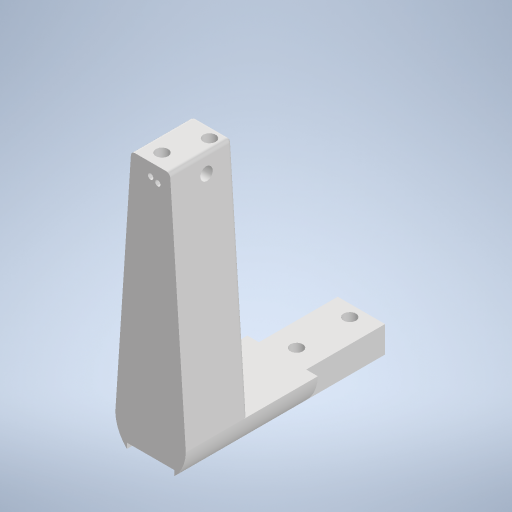
# Autodesk Inventor part: microstim_holder_bottom
Saved by Autodesk Inventor 2024 (Build 280153000, 153)
## iProperties
Created: 2023-05-03
Part Number: microstim_holder_bottom
Material: Generic
Document SubType Name: Modeling
Designer: Rober
Mass: 538.313 g
Surface Area: 676.575 cm^2
Volume: 538.313 cm^3
Density: 1 g/cm^3
Appearance: Default
Author: Rober
Autodesk Inventor part; units mm, degrees
ref_plane "YZ Plane" through (0, 0, 0) normal (1, 0, 0) x (0, 1, 0)
ref_plane "XZ Plane" through (0, 0, 0) normal (0, 1, 0) x (-1, 0, 0)
sketch "Sketch1" plane through (0, 0, 0) normal (0, 1, 0) x (-1, 0, 0)
  line L0 (3.05, -5.3255) -> (-3.05, -5.3255)
  line L1 (-3.05, -5.3255) -> (-3.05, 4.8245)
  line L2 (-3.05, 4.8245) -> (3.05, 4.8245)
  line L3 (3.05, 4.8245) -> (3.05, -5.3255)
  line L4 (0.925, 4.8245) -> (-0.925, 4.8245)
  line L5 (0.925, 4.8245) -> (0.925, -5.3255)
  line L6 (-0.925, 4.8245) -> (-0.925, -5.3255)
  circle A0 centre (0, 3.0245) radius 0.8
  circle A1 centre (0, -3.8255) radius 0.8
  line L7 (0, 4.8245) -> (0, -5.3255)
  line L8 (-3.05, 0) -> (3.05, 0)
  point P0 (0, 0)
  dimension "d13" = 6.1
  dimension "d44" = 1.85
  dimension "d45" = 2.125
  dimension "d46" = 1.6
  dimension "d47" = 1.6
  dimension "d128" = 6.85
  constraints: 18 end point, 9 point on line, 4 perpendicular, 3 midpoint, 2 centre point, 2 parallel, 1 horizontal
  measures "d13" distance of L0.start L0.end
  measures "d44" distance of L4.start L4.end
  measures "d45" distance from line of L3 L4.start
  measures "d46" diameter of A0
  measures "d47" diameter of A1
  measures "d128" distance of A0.centre A1.centre
extrude "Extrusion1" add sketch "Sketch1" along normal blind 3.4 contours L0 L5 L8 L3 | L0 L7 A1 L8 L5 | L8 L5 L2 L3 | L0 L6 L8 L7 A1 | L8 L7 A0 L2 L5 | L0 L1 L8 L6 | L8 L6 L2 L7 A0 | L8 L1 L2 L6
extrude "Extrusion6" add sketch "Sketch1" against normal blind 1 contours L0 L7 A1 L8 L5 | L0 L6 L8 L7 A1 | L8 L7 A0 L2 L5 | L8 L6 L2 L7 A0
sketch "Sketch13" plane through (-3.05, 3.4, 4.8245) normal (0, 0, 1) x (1, 0, 0)
  line L0 (0, 0) -> (0, -2.7)
  line L1 (0, -3.4) -> (0, 0) projected
  line L2 (0, -2.7) -> (6.1, -2.7)
  line L3 (6.1, -3.4) -> (6.1, 0) projected
  line L4 (6.1, 0) -> (6.1, -2.7)
  line L5 (0, 0) -> (6.1, 0)
  arc A0 (-1.4899, 0) -> (0, -3.4) centre (3.4689, 0.1465) ccw
  line L6 (-1.4899, 0) -> (12.0323, 0)
  line L7 (2.25, 0) -> (3.85, 0) projected
  line L8 (3.05, 0) -> (3.05, -3.4)
  line L9 (3.05, 0) -> (3.05, -3.4)
  arc A1 (6.1, -3.4) -> (7.5899, 0) centre (2.6311, 0.1465) ccw
  point P0 (6.1, -3.41)
  point P1 (7.5899, 0)
  dimension "d56" = 2.7
  constraints: 14 end point, 6 point on circle, 3 perpendicular, 2 centre point, 2 point on line, 2 symmetric about line, 1 collinear, 1 horizontal, 1 midpoint, 1 vertical, 1 other
  measures "d56" distance of L0.start L0.end
extrude "Extrusion8" add sketch "Sketch13" along normal blind 17
ref_plane "Work Plane3" through (-3.05, 3.4, 13.8245) normal (0, 0, 1) x (1, 0, 0)
sketch "Sketch29" plane through (-3.05, 3.4, 13.8245) normal (0, 0, 1) x (1, 0, 0)
  line L0 (3.85, -4.4) -> (2.25, -4.4) projected
  line L1 (3.05, -4.4) -> (3.05, 30.1)
  line L2 (5.55, 30.1) -> (3.05, 30.1)
  line L3 (3.05, 30.1) -> (0.55, 30.1)
  line L4 (5.55, 30.1) -> (7.5899, 0)
  line L5 (0.55, 30.1) -> (-1.4899, 0)
  line L6 (0, 0) -> (6.1, 0)
  line L7 (0, 0) -> (-1.4899, 0) projected
  line L8 (6.1, 0) -> (0, 0) projected
  line L9 (-1.4899, 0) -> (7.5899, 0)
  line L10 (-1.4899, 0) -> (7.5899, 0)
  point P0 (3.05, -3.4)
  point P1 (3.0506, 28.6)
  point P2 (3.05, 0)
  point P3 (3.05, 0)
  dimension "d137" = 34.5
  dimension "d156" = 2.5
  constraints: 17 end point, 3 collinear, 3 horizontal, 1 coincident, 1 midpoint, 1 vertical
  measures "d137" distance of L1.start L1.end
  measures "d156" distance of L2.start L1.end
extrude "Extrusion20" add sketch "Sketch29" along normal blind 8
fillet "Fillet6" radius 0.5 2 edges at (3.5199, 18.45, 13.8245) (-3.5199, 18.45, 13.8245)
sketch "Sketch24" plane through (-3.05, 0, -5.3255) normal (-1, 0, 0) x (0, 0, 1)
  circle A0 centre (22.5969, 31.2712) radius 0.8
  point P0 (5.3255, 0)
  point P1 (27.15, 0.7)
  dimension "d109" = 1.6
  constraints: 1 centre point
  measures "d109" diameter of A0
sketch "Sketch31" plane through (-3.05, 3.4, 13.8245) normal (0, 0, -1) x (-1, 0, 0)
  line L0 (-3.05, -3.4) -> (-3.05, 28.5)
  circle A0 centre (-3.05, 28.5) radius 0.355
  circle A1 centre (-3.9848, 28.2193) radius 0.355
  circle A2 centre (-3.9848, 28.2193) radius 0.3556 projected
  dimension "d145" = 31.9
  dimension "d147" = 0.71
  dimension "d155" = 0.71
  constraints: 2 centre point, 2 coincident, 2 end point, 1 vertical
  measures "d145" distance of L0.start L0.end
  measures "d147" diameter of A0
  measures "d155" diameter of A1
extrude "Extrusion22" cut sketch "Sketch31" against normal through all
fillet "Fillet7" radius 0.5 4 edges at (-2.5, 33.5, 18.0745) (2.3532, 33.5, 13.9709) (0, 33.5, 13.8245) (2.5, 33.5, 18.0745)
extrude "Extrusion24" cut sketch "Sketch24" against normal through all
sketch "Sketch35" plane through (-2.0327, 33.5, 21.8245) normal (0, 1, 0) x (1, 0, 0)
  circle A0 centre (3.1617, 6.4619) radius 0.8
  circle A1 centre (1.7036, 1.8035) radius 0.8
  point P0 (2.0327, 21.8245)
  dimension "d159" = 1.6
  dimension "d160" = 1.6
  constraints: 2 centre point
  measures "d159" diameter of A0
  measures "d160" diameter of A1
extrude "Extrusion25" cut sketch "Sketch35" against normal blind 1.5
equation "\"d13\" = base_width"
equation "\"d45\" = -0.5 * d44 + 0.5 * d13"
equation "\"d4\" = base_length"
equation "\"base_width\" = 6.1"
equation "\"base_length\" = 3.4"
equation "\"base_screw_diameter\" = 1.5"
equation "\"base_screw_spacing_edge\" = 8.5"
equation "\"multi_angle\" = 34deg"
body "Solid1"
